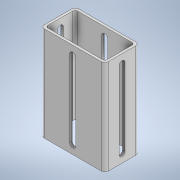
# Autodesk Inventor part: magazine-tower
Saved by Autodesk Inventor 2021 (Build 250183000, 183)
## iProperties
Created: 2024-03-19
Part Number: magazine-tower
Material: Generic
Document SubType Name: Modeling
Designer: 22hamfri
Density: 1 g/cm^3
Appearance: Default
Author: 22hamfri
Autodesk Inventor part; units mm, degrees
ref_plane "YZ Plane" through (0, 0, 0) normal (1, 0, 0) x (0, 1, 0)
ref_plane "XZ Plane" through (0, 0, 0) normal (0, 1, 0) x (-1, 0, 0)
ref_plane "XY Plane" through (0, 0, 0) normal (0, 0, 1) x (1, 0, 0)
sketch "Sketch1" plane through (0, 0, 0) normal (0, 1, 0) x (-1, 0, 0)
  line L0 (-25, 12.5) -> (25, 12.5)
  line L1 (25, 12.5) -> (25, -12.5)
  line L2 (25, -12.5) -> (-25, -12.5)
  line L3 (-25, -12.5) -> (-25, 12.5)
  line L4 (-25, 12.5) -> (25, -12.5) construction
  line L5 (25, 12.5) -> (-25, -12.5) construction
  line L6 (27, -14.5) -> (27, 14.5)
  line L7 (27, 14.5) -> (-27, 14.5)
  line L8 (-27, 14.5) -> (-27, -14.5)
  line L9 (-27, -14.5) -> (27, -14.5)
  point P0 (0, 0)
  dimension "d0" = 50
  dimension "d1" = 25
  dimension "d2" = 2
  constraints: 20 end point, 4 parallel, 2 midpoint, 2 perpendicular, 1 horizontal, 3 other
  measures "d0" distance between parallel lines of L3 L1
  measures "d1" distance between parallel lines of L2 L0
  measures "d2" distance between parallel lines of L1 L6
extrude "Extrusion1" add sketch "Sketch1" along normal blind 80
sketch "Sketch2" plane through (-27, 0, 14.5) normal (0, 0, 1) x (1, 0, 0)
  line L0 (0, 80) -> (54, 80) projected
  line L1 (27, 80) -> (27, 0)
  line L2 (24.5, 5) -> (24.5, 75)
  line L3 (24.5, 75) -> (29.5, 75)
  line L4 (29.5, 75) -> (29.5, 5)
  line L5 (29.5, 5) -> (24.5, 5)
  line L6 (24.5, 5) -> (29.5, 75) construction
  line L7 (24.5, 75) -> (29.5, 5) construction
  line L8 (0, 0) -> (0, 80) projected
  arc A0 (29.5, 72.5) -> (24.5, 72.5) centre (27, 72.5) ccw
  arc A1 (24.5, 7.5) -> (29.5, 7.5) centre (27, 7.5) ccw
  point P0 (27, 40)
  dimension "d5" = 5
  dimension "d6" = 5
  constraints: 14 end point, 6 point on line, 4 midpoint, 4 point on circle, 4 tangent, 3 parallel, 2 centre point, 1 perpendicular, 1 vertical
  measures "d5" distance between parallel lines of L4 L2
  measures "d6" distance between parallel lines of L3 L0
extrude "Extrusion2" cut sketch "Sketch2" against normal up to surface (29 mm away) contours A0 L4 A1 L1 | L1 A1 L2 A0
sketch "Sketch3" plane through (27, 0, 14.5) normal (1, 0, 0) x (0, 0, -1)
  line L0 (0, 80) -> (29, 80) projected
  line L1 (14.5, 80) -> (14.5, 0)
  line L2 (27, 0) -> (2, 0) projected
  line L3 (17, 5) -> (17, 75)
  line L4 (17, 75) -> (12, 75)
  line L5 (12, 75) -> (12, 5)
  line L6 (12, 5) -> (17, 5)
  line L7 (17, 5) -> (12, 75) construction
  line L8 (17, 75) -> (12, 5) construction
  line L9 (0, 0) -> (0, 80) projected
  arc A0 (17, 72.5) -> (12, 72.5) centre (14.5, 72.5) ccw
  arc A1 (12, 7.5) -> (17, 7.5) centre (14.5, 7.5) ccw
  point P0 (14.5, 40)
  dimension "d9" = 5
  dimension "d10" = 5
  constraints: 14 end point, 6 point on line, 4 midpoint, 4 point on circle, 4 tangent, 3 parallel, 2 centre point, 2 perpendicular
  measures "d9" distance between parallel lines of L3 L5
  measures "d10" distance between parallel lines of L4 L0
extrude "Extrusion3" cut sketch "Sketch3" against normal up to surface (54 mm away) contours A0 L3 A1 L1 | L1 A1 L5 A0
fillet "Fillet1" radius 2 4 edges at (-25, 40, -12.5) (-25, 40, 12.5) (25, 40, 12.5) (25, 40, -12.5)
fillet "Fillet2" radius 3 4 edges at (27, 40, 14.5) (27, 40, -14.5) (-27, 40, -14.5) (-27, 40, 14.5)
body "Solid1"
